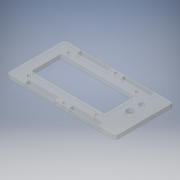
# Autodesk Inventor part: Interrupter_Top
Saved by Autodesk Inventor 2016 (Build 200138000, 138)
## iProperties
Created: 2018-05-24
Part Number: Interrupter_Top
Material: Polycarbonate, Clear
Document SubType Name: Modeling
Designer: Phil Erle
Density: 1.2 g/cm^3
Appearance: Polycarbonate - Clear
Author: Phil Erle
Autodesk Inventor part; units mm, degrees
ref_plane "YZ Plane" through (0, 0, 0) normal (1, 0, 0) x (0, 1, 0)
ref_plane "XZ Plane" through (0, 0, 0) normal (0, 1, 0) x (-1, 0, 0)
ref_plane "XY Plane" through (0, 0, 0) normal (0, 0, 1) x (1, 0, 0)
sketch "Sketch1" plane through (0, 0, 0) normal (0, 0, 1) x (1, 0, 0)
  line L0 (-75, -40) -> (75, -40)
  line L1 (75, -40) -> (75, 40)
  line L2 (75, 40) -> (-75, 40)
  line L3 (-75, 40) -> (-75, -40)
  line L4 (-75, -40) -> (75, 40) construction
  line L5 (75, -40) -> (-75, 40) construction
  point P0 (0, 0)
  dimension "d0" = 150
  dimension "d1" = 80
  constraints: 12 end point, 2 midpoint, 2 parallel, 1 horizontal, 1 perpendicular
  measures "d0" distance of L2.end L1.end
  measures "d1" distance of L1.end L0.end
extrude "Extrusion1" add sketch "Sketch1" along normal blind 5
sketch "Sketch4" plane through (0, 0, 5) normal (0, 0, 1) x (1, 0, 0)
  line L0 (-60, -20) -> (40, -20)
  line L1 (40, -20) -> (40, 20)
  line L2 (40, 20) -> (-60, 20)
  line L3 (-60, 20) -> (-60, -20)
  line L4 (-60, -20) -> (40, 20) construction
  line L5 (40, -20) -> (-60, 20) construction
  point P0 (0, 0)
  point P1 (-10, 0)
  point P2 (-10, 0)
  dimension "d8" = 100
  dimension "d9" = 40
  dimension "d10" = 10
  constraints: 12 end point, 3 midpoint, 2 parallel, 1 horizontal, 1 horizontal alignment, 1 perpendicular
  measures "d8" distance of L2.end L1.end
  measures "d9" distance of L1.end L0.end
  measures "d10" distance of point (0, 0) point (-10, 0)
extrude "Extrusion3" cut sketch "Sketch4" against normal through all
sketch "Sketch5" plane through (0, 0, 5) normal (0, 0, 1) x (1, 0, 0)
  line L0 (40, 20) -> (40, -20) projected
  point P0 (0, 0)
  point P1 (55, 0)
  dimension "d13" = 15
  constraints: 1 horizontal alignment
  measures "d13" distance from line of L0 point (55, 0)
hole "Hole1" at (55, 0, 5) direction (0, 0, -1) diameter 9 depth 8 tip angle 118 clearance for "Countersunk Flat Head Screw ISO 2009/7046" size "M8" standard "ISO"
sketch "Sketch6" plane through (0, 0, 5) normal (0, 0, 1) x (1, 0, 0)
  line L0 (-56.5, -27.5) -> (36.5, -27.5) construction
  line L1 (36.5, -27.5) -> (36.5, 27.5) construction
  line L2 (36.5, 27.5) -> (-56.5, 27.5) construction
  line L3 (-56.5, 27.5) -> (-56.5, -27.5) construction
  line L4 (-56.5, -27.5) -> (36.5, 27.5) construction
  line L5 (36.5, -27.5) -> (-56.5, 27.5) construction
  point P0 (0, 0)
  point P1 (-10, 0)
  point P2 (-10, 0)
  dimension "d21" = 93
  dimension "d22" = 55
  dimension "d23" = 10
  constraints: 12 end point, 4 coincident, 3 midpoint, 2 parallel, 1 horizontal, 1 horizontal alignment, 1 perpendicular
  measures "d21" distance of L1.end L2.end
  measures "d22" distance of L2.end L0.start
  measures "d23" distance of point (0, 0) point (-10, 0)
hole "Hole2" at (-56.5, 27.5, 5) at (36.5, 27.5, 5) at (36.5, -27.5, 5) at (-56.5, -27.5, 5) direction (0, 0, -1) diameter 3.4 depth 8 tip angle 118 clearance for "Countersunk Flat Head Screw ISO 2009/7046" size "M3" standard "ISO"
fillet "Fillet1" radius 2 4 edges at (-60, 20, 2.5) (-60, -20, 2.5) (40, -20, 2.5) (40, 20, 2.5)
fillet "Fillet2" radius 4 4 edges at (75, 40, 2.5) (-75, 40, 2.5) (75, -40, 2.5) (-75, -40, 2.5)
sketch "Sketch7" plane through (0, 0, 5) normal (0, 0, 1) x (1, 0, 0)
  line L0 (-50, 33) -> (50, 33) construction
  line L1 (50, 33) -> (50, 38) construction
  line L2 (50, 38) -> (-50, 38) construction
  line L3 (-50, 38) -> (-50, 33) construction
  line L4 (50, -38) -> (-50, -38) construction
  line L5 (-50, -38) -> (-50, -33) construction
  line L6 (-50, -33) -> (50, -33) construction
  line L7 (50, -33) -> (50, -38) construction
  line L8 (71, 40) -> (-71, 40) projected
  line L9 (-71, -40) -> (71, -40) projected
  line L10 (-50, 33) -> (-10, 33)
  line L11 (-10, 33) -> (-10, 38)
  line L12 (-10, 38) -> (-50, 38)
  line L13 (-50, 38) -> (-50, 33)
  line L14 (50, 33) -> (10, 33)
  line L15 (10, 33) -> (10, 38)
  line L16 (10, 38) -> (50, 38)
  line L17 (50, 38) -> (50, 33)
  line L18 (50, -38) -> (10, -38)
  line L19 (10, -38) -> (10, -33)
  line L20 (10, -33) -> (50, -33)
  line L21 (50, -33) -> (50, -38)
  line L22 (-50, -38) -> (-10, -38)
  line L23 (-10, -38) -> (-10, -33)
  line L24 (-10, -33) -> (-50, -33)
  line L25 (-50, -33) -> (-50, -38)
  point P0 (0, 0)
  point P1 (0, 38)
  dimension "d33" = 5
  dimension "d34" = 5
  dimension "d35" = 100
  dimension "d36" = 2
  dimension "d37" = 2
  dimension "d38" = 20
  dimension "d39" = 20
  dimension "d40" = 10
  dimension "d41" = 10
  constraints: 48 end point, 12 parallel, 6 horizontal, 6 perpendicular, 6 point on line, 1 midpoint, 1 vertical alignment
  measures "d33" distance of L2.end L0.start
  measures "d34" distance of L6.end L4.start
  measures "d35" distance of L1.end L2.end
  measures "d36" distance between parallel lines of L8 L2
  measures "d37" distance between parallel lines of L9 L4
  measures "d38" distance between parallel lines of L15 L11
  measures "d39" distance between parallel lines of L23 L19
  measures "d40" distance from line of point (0, 0) L11
  measures "d41" distance from line of point (0, 0) L23
extrude "Extrusion4" cut sketch "Sketch7" against normal blind 5
sketch "Sketch8" plane through (0, 0, 5) normal (0, 0, 1) x (1, 0, 0)
  line L0 (-50, -33) -> (-10, -33) projected
  line L1 (-10, 33) -> (-50, 33) projected
  point P0 (0, 0)
  point P1 (0, 35.5)
  point P2 (0, -35.5)
  dimension "d44" = 2.5
  dimension "d45" = 2.5
  constraints: 2 vertical alignment
  measures "d44" distance from line of point (0, -35.5) L0
  measures "d45" distance from line of L1 point (0, 35.5)
hole "Hole3" at (0, 35.5, 5) at (0, -35.5, 5) direction (0, 0, -1) diameter 3.4 depth 8 tip angle 118 clearance for "Countersunk Flat Head Screw ISO 2009/7046" size "M3" standard "ISO"
sketch "Sketch11" plane through (0, 0, 5) normal (0, 0, 1) x (1, 0, 0)
  circle A0 centre (55, 0) radius 4.5 projected
  point P0 (0, 0)
  point P1 (55, 16)
  dimension "d53" = 16
  constraints: 1 vertical alignment
  measures "d53" distance of point (55, 16) A0.centre
hole "Hole4" at (55, 16, 5) direction (0, 0, -1) diameter 6.2 depth 8 tip angle 118
equation "\"d40\" = 0.5 * d38"
equation "\"d41\" = 0.5 * d39"
body "Solid1"
